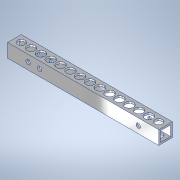
# Autodesk Inventor part: ロボット回転9ｘ9_1
Saved by Autodesk Inventor 2020.3 (Build 243373000, 373)
## iProperties
Created: 2020-07-04
Part Number: ロボット回転9ｘ9_1
Material: アルミニウム 6061
Document SubType Name: Modeling
Designer: totot
Density: 2.7 g/cm^3
Appearance: アルミニウム - フラット
Mass: 9.66735 g
Surface Area: 61.8564 cm^2
Volume: 3.5805 cm^3
Author: totot
Autodesk Inventor part; units mm, degrees
ref_plane "YZ Plane" through (0, 0, 0) normal (1, 0, 0) x (0, 1, 0)
ref_plane "XZ Plane" through (0, 0, 0) normal (0, 1, 0) x (-1, 0, 0)
ref_plane "XY Plane" through (0, 0, 0) normal (0, 0, 1) x (1, 0, 0)
sketch "スケッチ1" plane through (0, 0, 0) normal (1, 0, 0) x (0, 1, 0)
  line L0 (0, 0) -> (9, 0)
  line L1 (9, 0) -> (9, -9)
  line L2 (9, -9) -> (0, -9)
  line L3 (0, -9) -> (0, 0)
  line L4 (1.2, -1.2) -> (7.8, -1.2)
  line L5 (7.8, -1.2) -> (7.8, -7.8)
  line L6 (7.8, -7.8) -> (1.2, -7.8)
  line L7 (1.2, -7.8) -> (1.2, -1.2)
  dimension "d0" = 9
  dimension "d1" = 9
  dimension "d2" = 1.2
  dimension "d3" = 1.2
  dimension "d4" = 1.2
  dimension "d5" = 1.2
  constraints: 16 end point, 4 parallel, 2 horizontal, 2 perpendicular
  measures "d0" distance of L1.end L2.end
  measures "d1" distance of L0.end L1.end
  measures "d2" distance between parallel lines of L2 L6
  measures "d3" distance between parallel lines of L0 L4
  measures "d4" distance between parallel lines of L7 L3
  measures "d5" distance between parallel lines of L1 L5
extrude "押し出し1" add sketch "スケッチ1" along normal blind 99.5097
sketch "スケッチ2" plane through (0, 0, -9) normal (0, -1, 0) x (1, 0, 0)
  line L0 (0, 9) -> (0, 0) projected
  line L1 (99.5097, 9) -> (99.5097, 0) projected
  line L2 (0, 9) -> (99.5097, 9) projected
  point P0 (95.0097, 4.5)
  point P1 (4.5, 4.5)
  dimension "d8" = 4.5
  dimension "d9" = 4.5
  dimension "d10" = 4.5
  dimension "d11" = 4.5
  measures "d8" distance from line of point (4.5, 4.5) L0
  measures "d9" distance from line of L1 point (95.01, 4.5)
  measures "d10" distance from line of point (4.5, 4.5) L2
  measures "d11" distance from line of L2 point (95.01, 4.5)
hole "穴1" at (95.0097, 0, -4.5) at (4.5, 0, -4.5) direction (0, 1, 0) diameter 5 end through all
sketch "スケッチ3" plane through (0, 0, 0) normal (0, 0, 1) x (1, 0, 0)
  line L0 (0, 9) -> (0, 0) projected
  line L1 (0, 9) -> (99.5097, 9) projected
  line L2 (99.5097, 9) -> (99.5097, 0) projected
  point P0 (13.5, 4.5)
  point P1 (86.0097, 4.5)
  dimension "d19" = 13.5
  dimension "d20" = 4.5
  dimension "d21" = 4.5
  dimension "d22" = 13.5
  measures "d19" distance from line of point (13.5, 4.5) L0
  measures "d20" distance from line of point (13.5, 4.5) L1
  measures "d21" distance from line of point (86.01, 4.5) L1
  measures "d22" distance from line of point (86.01, 4.5) L2
hole "穴2" at (13.5, 4.5, 0) at (86.0097, 4.5, 0) direction (0, 0, -1) diameter 3 end through all
sketch "スケッチ5" plane through (0, 0, -9) normal (0, 0, -1) x (-1, 0, 0)
  line L0 (-99.5097, 0) -> (-99.5097, 9) projected
  line L1 (0, 9) -> (-99.5097, 9) projected
  point P0 (0, 0)
  point P1 (-21.0097, 4.5)
  dimension "d39" = 78.5
  dimension "d40" = 4.5
  measures "d39" distance from line of point (-21.01, 4.5) L0
  measures "d40" distance from line of point (-21.01, 4.5) L1
hole "穴4" at (21.0097, 4.5, -9) direction (0, 0, 1) diameter 3 end through all
sketch "スケッチ6" plane through (0, 0, -9) normal (0, -1, 0) x (1, 0, 0)
  circle A0 centre (95.0097, 4.5) radius 2.5 projected
  circle A1 centre (4.5, 4.5) radius 2.5 projected
  line L0 (4.5, 4.5) -> (95.0097, 4.5)
  point P0 (0, 9)
  point P1 (88.5447, 4.5)
  point P2 (82.0797, 4.5)
  point P3 (75.6147, 4.5)
  point P4 (69.1498, 4.5)
  point P5 (62.6848, 4.5)
  point P6 (56.2198, 4.5)
  point P7 (49.7548, 4.5)
  point P8 (43.2899, 4.5)
  point P9 (36.8249, 4.5)
  point P10 (30.3599, 4.5)
  point P11 (23.8949, 4.5)
  point P12 (17.43, 4.5)
  point P13 (10.965, 4.5)
  dimension "d48" = 90.5097
  dimension "d49" = 6.465
  dimension "d52" = 6.465
  constraints: 2 end point, 2 horizontal, 1 point on line, 12 other
  measures "d48" distance of L0.end L0.start
  measures "d49" distance of L0.end point (88.545, 4.5)
  measures "d52" distance of point (88.545, 4.5) point (82.08, 4.5)
hole "穴5" at (88.5447, 0, -4.5) at (82.0797, 0, -4.5) at (75.6147, 0, -4.5) at (69.1498, 0, -4.5) at (62.6848, 0, -4.5) at (56.2198, 0, -4.5) at (49.7548, 0, -4.5) at (43.2899, 0, -4.5) at (36.8249, 0, -4.5) at (30.3599, 0, -4.5) at (23.8949, 0, -4.5) at (17.43, 0, -4.5) at (10.965, 0, -4.5) direction (0, 1, 0) diameter 5.5 end through all
sketch "スケッチ7" plane through (0, 0, -9) normal (0, 0, -1) x (-1, 0, 0)
  line L0 (0, 9) -> (-99.5097, 9) projected
  circle A0 centre (-13.5, 4.5) radius 1.5 projected
  line L1 (0, 0) -> (0, 9) projected
  line L2 (-99.5097, 0) -> (-99.5097, 9) projected
  circle A1 centre (-86.0097, 4.5) radius 1.5 projected
  circle A2 centre (-21.0097, 4.5) radius 1.5 projected
  line L3 (-86.0097, 4.5) -> (-21.0097, 4.5)
  point P0 (-92.7597, 4.5)
  point P1 (-6.75, 4.5)
  point P2 (-79.5097, 4.5)
  point P3 (-73.0097, 4.5)
  point P4 (-66.5097, 4.5)
  point P5 (-60.0097, 4.5)
  point P6 (-53.5097, 4.5)
  point P7 (-47.0097, 4.5)
  point P8 (-40.5097, 4.5)
  point P9 (-34.0097, 4.5)
  point P10 (-27.5097, 4.5)
  dimension "d64" = 4.5
  dimension "d65" = 4.5
  dimension "d68" = 13.5
  dimension "d69" = 6.75
  dimension "d70" = 13.5
  dimension "d71" = 6.75
  dimension "d72" = 65
  dimension "d73" = 6.5
  dimension "d76" = 6.5
  constraints: 2 end point, 2 horizontal, 1 point on line, 8 other
  measures "d64" distance from line of point (-92.76, 4.5) L0
  measures "d65" distance from line of point (-6.75, 4.5) L0
  measures "d68" distance from line of L2 L3.start
  measures "d69" distance of L3.start point (-92.76, 4.5)
  measures "d70" distance from line of L1 A0.centre
  measures "d71" distance of point (-6.75, 4.5) A0.centre
  measures "d72" distance of L3.end L3.start
  measures "d73" distance of point (-79.51, 4.5) L3.start
  measures "d76" distance of point (-79.51, 4.5) point (-73.01, 4.5)
hole "穴6" at (92.7597, 4.5, -9) at (6.75, 4.5, -9) at (79.5097, 4.5, -9) at (73.0097, 4.5, -9) at (66.5097, 4.5, -9) at (60.0097, 4.5, -9) at (53.5097, 4.5, -9) at (47.0097, 4.5, -9) at (40.5097, 4.5, -9) at (34.0097, 4.5, -9) at (27.5097, 4.5, -9) direction (0, 0, 1) diameter 5.5 end through all
equation "\"d3\" = d2"
equation "\"d4\" = d2"
equation "\"d5\" = d4"
equation "\"d9\" = d8"
equation "\"d11\" = d10"
equation "\"d49\" = 0.0714286 * d48"
equation "\"d52\" = d49"
equation "\"d69\" = 0.5 * d68"
equation "\"d71\" = 0.5 * d70"
equation "\"d73\" = 0.1 * d72"
equation "\"d76\" = d73"
